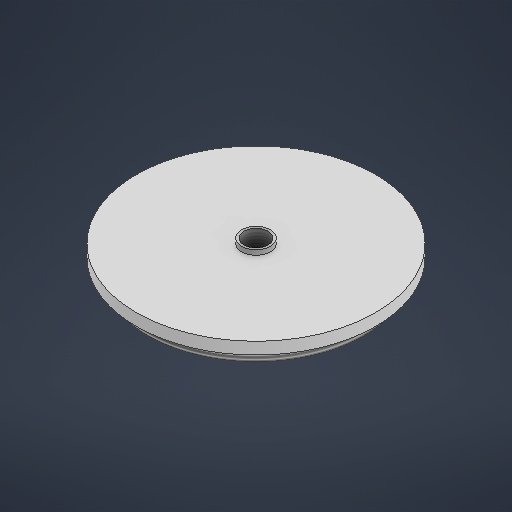
# Autodesk Inventor part: Pieza3
Saved by Autodesk Inventor 2026.1 (Build 301233000, 233)
## iProperties
Created: 2025-09-19
Part Number: Pieza3
Material: Genérico
Document SubType Name: Modeling
Designer: Usuario
Density: 1 g/cm^3
Appearance: Valor por defecto
Author: Usuario
Autodesk Inventor part; units mm, degrees
ref_plane "YZ Plane" through (0, 0, 0) normal (1, 0, 0) x (0, 1, 0)
ref_plane "XZ Plane" through (0, 0, 0) normal (0, 1, 0) x (-1, 0, 0)
ref_plane "XY Plane" through (0, 0, 0) normal (0, 0, 1) x (1, 0, 0)
sketch "Boceto1" plane through (0, 0, 0) normal (0, 1, 0) x (-1, 0, 0)
  line L0 (0, 0) -> (100, 0) construction
  line L1 (100, 0) -> (100, -100) construction
  line L2 (100, -100) -> (0, -100) construction
  line L3 (0, -100) -> (0, 0) construction
  line L4 (100, -100) -> (0, 0) construction
  line L5 (100, 0) -> (0, -100) construction
  circle A0 centre (50, -50) radius 50
  dimension "d0" = 100
  dimension "d1" = 100
  dimension "d2" = 100
  constraints: 12 end point, 2 parallel, 1 centre point, 1 horizontal, 1 midpoint, 1 perpendicular
  measures "d0" distance of L1.end L2.end
  measures "d1" distance of L0.end L1.end
  measures "d2" diameter of A0
extrude "Extrusión1" add sketch "Boceto1" along normal blind 5
sketch "Boceto2" plane through (-50, 0, -50) normal (0, -1, 0) x (1, 0, 0)
  circle A0 centre (0, 0) radius 45
  point P0 (50, 50)
  dimension "d5" = 90
  constraints: 1 centre point
  measures "d5" diameter of A0
extrude "Extrusión2" add sketch "Boceto2" along normal blind 6
thread "Rosca1" size "M80x1.5" class "6g" standard "ANSI Metric M Profile" length 6
sketch "Boceto3" plane through (-50, 5, -50) normal (0, 1, 0) x (1, 0, 0)
  circle A0 centre (0, 0) radius 6
  point P0 (50, -50)
  dimension "d10" = 12
  constraints: 1 centre point
  measures "d10" diameter of A0
extrude "Extrusión3" add sketch "Boceto3" along normal blind 2
sketch "Boceto4" plane through (-50, 7, -50) normal (0, 1, 0) x (1, 0, 0)
  circle A0 centre (0, 0) radius 5
  point P0 (50, -50)
  dimension "d13" = 10
  constraints: 1 centre point
  measures "d13" diameter of A0
extrude "Extrusión4" cut sketch "Boceto4" against normal through all
thread "Rosca2" size "M9x1.25" class "6H" standard "ANSI Metric M Profile" full length
